Autodesk Fusion 360 part; units mm, degrees
(part 7 of 9)
sketch "草图25" plane through (0, -82, 0) normal (0, 1, 0) x (-1, 0, 0)
  line L0 (41, 0) -> (116, 0)
  line L1 (116, 0) -> (116, 140)
  line L2 (116, 140) -> (41, 140)
  line L3 (41, 140) -> (41, 0)
  line L4 (53.0801, 20.799) -> (48.75, 18.299)
  line L5 (48.75, 18.299) -> (48.75, 13.299)
  line L6 (48.75, 13.299) -> (53.0801, 10.799)
  line L7 (53.0801, 10.799) -> (57.4103, 13.299)
  line L8 (57.4103, 13.299) -> (57.4103, 18.299)
  line L9 (57.4103, 18.299) -> (53.0801, 20.799)
  line L10 (63.2404, 20.799) -> (58.9103, 18.299)
  line L11 (58.9103, 18.299) -> (58.9103, 13.299)
  line L12 (58.9103, 13.299) -> (63.2404, 10.799)
  line L13 (63.2404, 10.799) -> (67.5705, 13.299)
  line L14 (67.5705, 13.299) -> (67.5705, 18.299)
  line L15 (67.5705, 18.299) -> (63.2404, 20.799)
  line L16 (73.4006, 20.799) -> (69.0705, 18.299)
  line L17 (69.0705, 18.299) -> (69.0705, 13.299)
  line L18 (69.0705, 13.299) -> (73.4006, 10.799)
  line L19 (73.4006, 10.799) -> (77.7308, 13.299)
  line L20 (77.7308, 13.299) -> (77.7308, 18.299)
  line L21 (77.7308, 18.299) -> (73.4006, 20.799)
  line L22 (83.5609, 20.799) -> (79.2308, 18.299)
  line L23 (79.2308, 18.299) -> (79.2308, 13.299)
  line L24 (79.2308, 13.299) -> (83.5609, 10.799)
  line L25 (83.5609, 10.799) -> (87.891, 13.299)
  line L26 (87.891, 13.299) -> (87.891, 18.299)
  line L27 (87.891, 18.299) -> (83.5609, 20.799)
  line L28 (93.7211, 20.799) -> (89.391, 18.299)
  line L29 (89.391, 18.299) -> (89.391, 13.299)
  line L30 (89.391, 13.299) -> (93.7211, 10.799)
  line L31 (93.7211, 10.799) -> (98.0513, 13.299)
  line L32 (98.0513, 13.299) -> (98.0513, 18.299)
  line L33 (98.0513, 18.299) -> (93.7211, 20.799)
  line L34 (103.8814, 20.799) -> (99.5513, 18.299)
  line L35 (99.5513, 18.299) -> (99.5513, 13.299)
  line L36 (99.5513, 13.299) -> (103.8814, 10.799)
  line L37 (103.8814, 10.799) -> (108.2115, 13.299)
  line L38 (108.2115, 13.299) -> (108.2115, 18.299)
  line L39 (108.2115, 18.299) -> (103.8814, 20.799)
  line L40 (48, 29.5981) -> (43.6699, 27.0981)
  line L41 (43.6699, 27.0981) -> (43.6699, 22.0981)
  line L42 (43.6699, 22.0981) -> (48, 19.5981)
  line L43 (48, 19.5981) -> (52.3301, 22.0981)
  line L44 (52.3301, 22.0981) -> (52.3301, 27.0981)
  line L45 (52.3301, 27.0981) -> (48, 29.5981)
  line L46 (58.1603, 29.5981) -> (53.8301, 27.0981)
  line L47 (53.8301, 27.0981) -> (53.8301, 22.0981)
  line L48 (53.8301, 22.0981) -> (58.1603, 19.5981)
  line L49 (58.1603, 19.5981) -> (62.4904, 22.0981)
  line L50 (62.4904, 22.0981) -> (62.4904, 27.0981)
  line L51 (62.4904, 27.0981) -> (58.1603, 29.5981)
  line L52 (68.3205, 29.5981) -> (63.9904, 27.0981)
  line L53 (63.9904, 27.0981) -> (63.9904, 22.0981)
  line L54 (63.9904, 22.0981) -> (68.3205, 19.5981)
  line L55 (68.3205, 19.5981) -> (72.6506, 22.0981)
  line L56 (72.6506, 22.0981) -> (72.6506, 27.0981)
  line L57 (72.6506, 27.0981) -> (68.3205, 29.5981)
  line L58 (78.4808, 29.5981) -> (74.1506, 27.0981)
  line L59 (74.1506, 27.0981) -> (74.1506, 22.0981)
  line L60 (74.1506, 22.0981) -> (78.4808, 19.5981)
  line L61 (78.4808, 19.5981) -> (82.8109, 22.0981)
  line L62 (82.8109, 22.0981) -> (82.8109, 27.0981)
  line L63 (82.8109, 27.0981) -> (78.4808, 29.5981)
  line L64 (88.641, 29.5981) -> (84.3109, 27.0981)
  line L65 (84.3109, 27.0981) -> (84.3109, 22.0981)
  line L66 (84.3109, 22.0981) -> (88.641, 19.5981)
  line L67 (88.641, 19.5981) -> (92.9711, 22.0981)
  line L68 (92.9711, 22.0981) -> (92.9711, 27.0981)
  line L69 (92.9711, 27.0981) -> (88.641, 29.5981)
  line L70 (98.8013, 29.5981) -> (94.4711, 27.0981)
  line L71 (94.4711, 27.0981) -> (94.4711, 22.0981)
  line L72 (94.4711, 22.0981) -> (98.8013, 19.5981)
  line L73 (98.8013, 19.5981) -> (103.1314, 22.0981)
  line L74 (103.1314, 22.0981) -> (103.1314, 27.0981)
  line L75 (103.1314, 27.0981) -> (98.8013, 29.5981)
  line L76 (108.9615, 29.5981) -> (104.6314, 27.0981)
  line L77 (104.6314, 27.0981) -> (104.6314, 22.0981)
  line L78 (104.6314, 22.0981) -> (108.9615, 19.5981)
  line L79 (108.9615, 19.5981) -> (113.2917, 22.0981)
  line L80 (113.2917, 22.0981) -> (113.2917, 27.0981)
  line L81 (113.2917, 27.0981) -> (108.9615, 29.5981)
  line L82 (53.0801, 38.3971) -> (48.75, 35.8971)
  line L83 (48.75, 35.8971) -> (48.75, 30.8971)
  line L84 (48.75, 30.8971) -> (53.0801, 28.3971)
  line L85 (53.0801, 28.3971) -> (57.4103, 30.8971)
  line L86 (57.4103, 30.8971) -> (57.4103, 35.8971)
  line L87 (57.4103, 35.8971) -> (53.0801, 38.3971)
  line L88 (63.2404, 38.3971) -> (58.9103, 35.8971)
  line L89 (58.9103, 35.8971) -> (58.9103, 30.8971)
  line L90 (58.9103, 30.8971) -> (63.2404, 28.3971)
  line L91 (63.2404, 28.3971) -> (67.5705, 30.8971)
  line L92 (67.5705, 30.8971) -> (67.5705, 35.8971)
  line L93 (67.5705, 35.8971) -> (63.2404, 38.3971)
  line L94 (73.4006, 38.3971) -> (69.0705, 35.8971)
  line L95 (69.0705, 35.8971) -> (69.0705, 30.8971)
  line L96 (69.0705, 30.8971) -> (73.4006, 28.3971)
  line L97 (73.4006, 28.3971) -> (77.7308, 30.8971)
  line L98 (77.7308, 30.8971) -> (77.7308, 35.8971)
  line L99 (77.7308, 35.8971) -> (73.4006, 38.3971)
  line L100 (83.5609, 38.3971) -> (79.2308, 35.8971)
  line L101 (79.2308, 35.8971) -> (79.2308, 30.8971)
  line L102 (79.2308, 30.8971) -> (83.5609, 28.3971)
  line L103 (83.5609, 28.3971) -> (87.891, 30.8971)
  line L104 (87.891, 30.8971) -> (87.891, 35.8971)
  line L105 (87.891, 35.8971) -> (83.5609, 38.3971)
  line L106 (93.7211, 38.3971) -> (89.391, 35.8971)
  line L107 (89.391, 35.8971) -> (89.391, 30.8971)
  line L108 (89.391, 30.8971) -> (93.7211, 28.3971)
  line L109 (93.7211, 28.3971) -> (98.0513, 30.8971)
  line L110 (98.0513, 30.8971) -> (98.0513, 35.8971)
  line L111 (98.0513, 35.8971) -> (93.7211, 38.3971)
  line L112 (103.8814, 38.3971) -> (99.5513, 35.8971)
  line L113 (99.5513, 35.8971) -> (99.5513, 30.8971)
  line L114 (99.5513, 30.8971) -> (103.8814, 28.3971)
  line L115 (103.8814, 28.3971) -> (108.2115, 30.8971)
  line L116 (108.2115, 30.8971) -> (108.2115, 35.8971)
  line L117 (108.2115, 35.8971) -> (103.8814, 38.3971)
  line L118 (48, 47.1962) -> (43.6699, 44.6962)
  line L119 (43.6699, 44.6962) -> (43.6699, 39.6962)
  line L120 (43.6699, 39.6962) -> (48, 37.1962)
  line L121 (48, 37.1962) -> (52.3301, 39.6962)
  line L122 (52.3301, 39.6962) -> (52.3301, 44.6962)
  line L123 (52.3301, 44.6962) -> (48, 47.1962)
  line L124 (58.1603, 47.1962) -> (53.8301, 44.6962)
  line L125 (53.8301, 44.6962) -> (53.8301, 39.6962)
  line L126 (53.8301, 39.6962) -> (58.1603, 37.1962)
  line L127 (58.1603, 37.1962) -> (62.4904, 39.6962)
  line L128 (62.4904, 39.6962) -> (62.4904, 44.6962)
  line L129 (62.4904, 44.6962) -> (58.1603, 47.1962)
  line L130 (68.3205, 47.1962) -> (63.9904, 44.6962)
  line L131 (63.9904, 44.6962) -> (63.9904, 39.6962)
  line L132 (63.9904, 39.6962) -> (68.3205, 37.1962)
  line L133 (68.3205, 37.1962) -> (72.6506, 39.6962)
  line L134 (72.6506, 39.6962) -> (72.6506, 44.6962)
  line L135 (72.6506, 44.6962) -> (68.3205, 47.1962)
  line L136 (78.4808, 47.1962) -> (74.1506, 44.6962)
  line L137 (74.1506, 44.6962) -> (74.1506, 39.6962)
  line L138 (74.1506, 39.6962) -> (78.4808, 37.1962)
  line L139 (78.4808, 37.1962) -> (82.8109, 39.6962)
  line L140 (82.8109, 39.6962) -> (82.8109, 44.6962)
  line L141 (82.8109, 44.6962) -> (78.4808, 47.1962)
  line L142 (88.641, 47.1962) -> (84.3109, 44.6962)
  line L143 (84.3109, 44.6962) -> (84.3109, 39.6962)
  line L144 (84.3109, 39.6962) -> (88.641, 37.1962)
  line L145 (88.641, 37.1962) -> (92.9711, 39.6962)
  line L146 (92.9711, 39.6962) -> (92.9711, 44.6962)
  line L147 (92.9711, 44.6962) -> (88.641, 47.1962)
  line L148 (98.8013, 47.1962) -> (94.4711, 44.6962)
  line L149 (94.4711, 44.6962) -> (94.4711, 39.6962)
  line L150 (94.4711, 39.6962) -> (98.8013, 37.1962)
  line L151 (98.8013, 37.1962) -> (103.1314, 39.6962)
  line L152 (103.1314, 39.6962) -> (103.1314, 44.6962)
  line L153 (103.1314, 44.6962) -> (98.8013, 47.1962)
  line L154 (108.9615, 47.1962) -> (104.6314, 44.6962)
  line L155 (104.6314, 44.6962) -> (104.6314, 39.6962)
  line L156 (104.6314, 39.6962) -> (108.9615, 37.1962)
  line L157 (108.9615, 37.1962) -> (113.2917, 39.6962)
  line L158 (113.2917, 39.6962) -> (113.2917, 44.6962)
  line L159 (113.2917, 44.6962) -> (108.9615, 47.1962)
  line L160 (53.0801, 55.9952) -> (48.75, 53.4952)
  line L161 (48.75, 53.4952) -> (48.75, 48.4952)
  line L162 (48.75, 48.4952) -> (53.0801, 45.9952)
  line L163 (53.0801, 45.9952) -> (57.4103, 48.4952)
  line L164 (57.4103, 48.4952) -> (57.4103, 53.4952)
  line L165 (57.4103, 53.4952) -> (53.0801, 55.9952)
  line L166 (63.2404, 55.9952) -> (58.9103, 53.4952)
  line L167 (58.9103, 53.4952) -> (58.9103, 48.4952)
  line L168 (58.9103, 48.4952) -> (63.2404, 45.9952)
  line L169 (63.2404, 45.9952) -> (67.5705, 48.4952)
  line L170 (67.5705, 48.4952) -> (67.5705, 53.4952)
  line L171 (67.5705, 53.4952) -> (63.2404, 55.9952)
  line L172 (73.4006, 55.9952) -> (69.0705, 53.4952)
  line L173 (69.0705, 53.4952) -> (69.0705, 48.4952)
  line L174 (69.0705, 48.4952) -> (73.4006, 45.9952)
  line L175 (73.4006, 45.9952) -> (77.7308, 48.4952)
  line L176 (77.7308, 48.4952) -> (77.7308, 53.4952)
  line L177 (77.7308, 53.4952) -> (73.4006, 55.9952)
  line L178 (83.5609, 55.9952) -> (79.2308, 53.4952)
  line L179 (79.2308, 53.4952) -> (79.2308, 48.4952)
  line L180 (79.2308, 48.4952) -> (83.5609, 45.9952)
  line L181 (83.5609, 45.9952) -> (87.891, 48.4952)
  line L182 (87.891, 48.4952) -> (87.891, 53.4952)
  line L183 (87.891, 53.4952) -> (83.5609, 55.9952)
  line L184 (93.7211, 55.9952) -> (89.391, 53.4952)
  line L185 (89.391, 53.4952) -> (89.391, 48.4952)
  line L186 (89.391, 48.4952) -> (93.7211, 45.9952)
  line L187 (93.7211, 45.9952) -> (98.0513, 48.4952)
  line L188 (98.0513, 48.4952) -> (98.0513, 53.4952)
  line L189 (98.0513, 53.4952) -> (93.7211, 55.9952)
  line L190 (103.8814, 55.9952) -> (99.5513, 53.4952)
  line L191 (99.5513, 53.4952) -> (99.5513, 48.4952)
  line L192 (99.5513, 48.4952) -> (103.8814, 45.9952)
  line L193 (103.8814, 45.9952) -> (108.2115, 48.4952)
  line L194 (108.2115, 48.4952) -> (108.2115, 53.4952)
  line L195 (108.2115, 53.4952) -> (103.8814, 55.9952)
  line L196 (48, 64.7942) -> (43.6699, 62.2942)
  line L197 (43.6699, 62.2942) -> (43.6699, 57.2942)
  line L198 (43.6699, 57.2942) -> (48, 54.7942)
  line L199 (48, 54.7942) -> (52.3301, 57.2942)
  line L200 (52.3301, 57.2942) -> (52.3301, 62.2942)
  line L201 (52.3301, 62.2942) -> (48, 64.7942)
  line L202 (58.1603, 64.7942) -> (53.8301, 62.2942)
  line L203 (53.8301, 62.2942) -> (53.8301, 57.2942)
  line L204 (53.8301, 57.2942) -> (58.1603, 54.7942)
  line L205 (58.1603, 54.7942) -> (62.4904, 57.2942)
  line L206 (62.4904, 57.2942) -> (62.4904, 62.2942)
  line L207 (62.4904, 62.2942) -> (58.1603, 64.7942)
  line L208 (68.3205, 64.7942) -> (63.9904, 62.2942)
  line L209 (63.9904, 62.2942) -> (63.9904, 57.2942)
  line L210 (63.9904, 57.2942) -> (68.3205, 54.7942)
  line L211 (68.3205, 54.7942) -> (72.6506, 57.2942)
  line L212 (72.6506, 57.2942) -> (72.6506, 62.2942)
  line L213 (72.6506, 62.2942) -> (68.3205, 64.7942)
  line L214 (78.4808, 64.7942) -> (74.1506, 62.2942)
  line L215 (74.1506, 62.2942) -> (74.1506, 57.2942)
  line L216 (74.1506, 57.2942) -> (78.4808, 54.7942)
  line L217 (78.4808, 54.7942) -> (82.8109, 57.2942)
  line L218 (82.8109, 57.2942) -> (82.8109, 62.2942)
  line L219 (82.8109, 62.2942) -> (78.4808, 64.7942)
  line L220 (88.641, 64.7942) -> (84.3109, 62.2942)
  line L221 (84.3109, 62.2942) -> (84.3109, 57.2942)
  line L222 (84.3109, 57.2942) -> (88.641, 54.7942)
  line L223 (88.641, 54.7942) -> (92.9711, 57.2942)
  line L224 (92.9711, 57.2942) -> (92.9711, 62.2942)
  line L225 (92.9711, 62.2942) -> (88.641, 64.7942)
  line L226 (98.8013, 64.7942) -> (94.4711, 62.2942)
  line L227 (94.4711, 62.2942) -> (94.4711, 57.2942)
  line L228 (94.4711, 57.2942) -> (98.8013, 54.7942)
  line L229 (98.8013, 54.7942) -> (103.1314, 57.2942)
  line L230 (103.1314, 57.2942) -> (103.1314, 62.2942)
  line L231 (103.1314, 62.2942) -> (98.8013, 64.7942)
  line L232 (108.9615, 64.7942) -> (104.6314, 62.2942)
  line L233 (104.6314, 62.2942) -> (104.6314, 57.2942)
  line L234 (104.6314, 57.2942) -> (108.9615, 54.7942)
  line L235 (108.9615, 54.7942) -> (113.2917, 57.2942)
  line L236 (113.2917, 57.2942) -> (113.2917, 62.2942)
  line L237 (113.2917, 62.2942) -> (108.9615, 64.7942)
  line L238 (53.0801, 73.5933) -> (48.75, 71.0933)
  line L239 (48.75, 71.0933) -> (48.75, 66.0933)
  line L240 (48.75, 66.0933) -> (53.0801, 63.5933)
  line L241 (53.0801, 63.5933) -> (57.4103, 66.0933)
  line L242 (57.4103, 66.0933) -> (57.4103, 71.0933)
  line L243 (57.4103, 71.0933) -> (53.0801, 73.5933)
  line L244 (63.2404, 73.5933) -> (58.9103, 71.0933)
  line L245 (58.9103, 71.0933) -> (58.9103, 66.0933)
  line L246 (58.9103, 66.0933) -> (63.2404, 63.5933)
  line L247 (63.2404, 63.5933) -> (67.5705, 66.0933)
  line L248 (67.5705, 66.0933) -> (67.5705, 71.0933)
  line L249 (67.5705, 71.0933) -> (63.2404, 73.5933)
  line L250 (73.4006, 73.5933) -> (69.0705, 71.0933)
  line L251 (69.0705, 71.0933) -> (69.0705, 66.0933)
  line L252 (69.0705, 66.0933) -> (73.4006, 63.5933)
  line L253 (73.4006, 63.5933) -> (77.7308, 66.0933)
  line L254 (77.7308, 66.0933) -> (77.7308, 71.0933)
  line L255 (77.7308, 71.0933) -> (73.4006, 73.5933)
  line L256 (83.5609, 73.5933) -> (79.2308, 71.0933)
  line L257 (79.2308, 71.0933) -> (79.2308, 66.0933)
  line L258 (79.2308, 66.0933) -> (83.5609, 63.5933)
  line L259 (83.5609, 63.5933) -> (87.891, 66.0933)
  line L260 (87.891, 66.0933) -> (87.891, 71.0933)
  line L261 (87.891, 71.0933) -> (83.5609, 73.5933)
  line L262 (93.7211, 73.5933) -> (89.391, 71.0933)
  line L263 (89.391, 71.0933) -> (89.391, 66.0933)
  line L264 (89.391, 66.0933) -> (93.7211, 63.5933)
  line L265 (93.7211, 63.5933) -> (98.0513, 66.0933)
  line L266 (98.0513, 66.0933) -> (98.0513, 71.0933)
  line L267 (98.0513, 71.0933) -> (93.7211, 73.5933)
  line L268 (103.8814, 73.5933) -> (99.5513, 71.0933)
  line L269 (99.5513, 71.0933) -> (99.5513, 66.0933)
  line L270 (99.5513, 66.0933) -> (103.8814, 63.5933)
  line L271 (103.8814, 63.5933) -> (108.2115, 66.0933)
  line L272 (108.2115, 66.0933) -> (108.2115, 71.0933)
  line L273 (108.2115, 71.0933) -> (103.8814, 73.5933)
  line L274 (48, 82.3923) -> (43.6699, 79.8923)
  line L275 (43.6699, 79.8923) -> (43.6699, 74.8923)
  line L276 (43.6699, 74.8923) -> (48, 72.3923)
  line L277 (48, 72.3923) -> (52.3301, 74.8923)
  line L278 (52.3301, 74.8923) -> (52.3301, 79.8923)
  line L279 (52.3301, 79.8923) -> (48, 82.3923)
  line L280 (58.1603, 82.3923) -> (53.8301, 79.8923)
  line L281 (53.8301, 79.8923) -> (53.8301, 74.8923)
  line L282 (53.8301, 74.8923) -> (58.1603, 72.3923)
  line L283 (58.1603, 72.3923) -> (62.4904, 74.8923)
  line L284 (62.4904, 74.8923) -> (62.4904, 79.8923)
  line L285 (62.4904, 79.8923) -> (58.1603, 82.3923)
  line L286 (68.3205, 82.3923) -> (63.9904, 79.8923)
  line L287 (63.9904, 79.8923) -> (63.9904, 74.8923)
  line L288 (63.9904, 74.8923) -> (68.3205, 72.3923)
  line L289 (68.3205, 72.3923) -> (72.6506, 74.8923)
  line L290 (72.6506, 74.8923) -> (72.6506, 79.8923)
  line L291 (72.6506, 79.8923) -> (68.3205, 82.3923)
  line L292 (78.4808, 82.3923) -> (74.1506, 79.8923)
  line L293 (74.1506, 79.8923) -> (74.1506, 74.8923)
  line L294 (74.1506, 74.8923) -> (78.4808, 72.3923)
  line L295 (78.4808, 72.3923) -> (82.8109, 74.8923)
  line L296 (82.8109, 74.8923) -> (82.8109, 79.8923)
  line L297 (82.8109, 79.8923) -> (78.4808, 82.3923)
  line L298 (88.641, 82.3923) -> (84.3109, 79.8923)
  line L299 (84.3109, 79.8923) -> (84.3109, 74.8923)
  line L300 (84.3109, 74.8923) -> (88.641, 72.3923)
  line L301 (88.641, 72.3923) -> (92.9711, 74.8923)
  line L302 (92.9711, 74.8923) -> (92.9711, 79.8923)
  line L303 (92.9711, 79.8923) -> (88.641, 82.3923)
  line L304 (98.8013, 82.3923) -> (94.4711, 79.8923)
  line L305 (94.4711, 79.8923) -> (94.4711, 74.8923)
  line L306 (94.4711, 74.8923) -> (98.8013, 72.3923)
  line L307 (98.8013, 72.3923) -> (103.1314, 74.8923)
  line L308 (103.1314, 74.8923) -> (103.1314, 79.8923)
  line L309 (103.1314, 79.8923) -> (98.8013, 82.3923)
  line L310 (108.9615, 82.3923) -> (104.6314, 79.8923)
  line L311 (104.6314, 79.8923) -> (104.6314, 74.8923)
  line L312 (104.6314, 74.8923) -> (108.9615, 72.3923)
  line L313 (108.9615, 72.3923) -> (113.2917, 74.8923)
  line L314 (113.2917, 74.8923) -> (113.2917, 79.8923)
  line L315 (113.2917, 79.8923) -> (108.9615, 82.3923)
  line L316 (53.0801, 91.1913) -> (48.75, 88.6913)
  line L317 (48.75, 88.6913) -> (48.75, 83.6913)
  line L318 (48.75, 83.6913) -> (53.0801, 81.1913)
  line L319 (53.0801, 81.1913) -> (57.4103, 83.6913)
  line L320 (57.4103, 83.6913) -> (57.4103, 88.6913)
  line L321 (57.4103, 88.6913) -> (53.0801, 91.1913)
  line L322 (63.2404, 91.1913) -> (58.9103, 88.6913)
  line L323 (58.9103, 88.6913) -> (58.9103, 83.6913)
  line L324 (58.9103, 83.6913) -> (63.2404, 81.1913)
  line L325 (63.2404, 81.1913) -> (67.5705, 83.6913)
  line L326 (67.5705, 83.6913) -> (67.5705, 88.6913)
  line L327 (67.5705, 88.6913) -> (63.2404, 91.1913)
  line L328 (73.4006, 91.1913) -> (69.0705, 88.6913)
  line L329 (69.0705, 88.6913) -> (69.0705, 83.6913)
  line L330 (69.0705, 83.6913) -> (73.4006, 81.1913)
  line L331 (73.4006, 81.1913) -> (77.7308, 83.6913)
  line L332 (77.7308, 83.6913) -> (77.7308, 88.6913)
  line L333 (77.7308, 88.6913) -> (73.4006, 91.1913)
  line L334 (83.5609, 91.1913) -> (79.2308, 88.6913)
  line L335 (79.2308, 88.6913) -> (79.2308, 83.6913)
  line L336 (79.2308, 83.6913) -> (83.5609, 81.1913)
  line L337 (83.5609, 81.1913) -> (87.891, 83.6913)
  line L338 (87.891, 83.6913) -> (87.891, 88.6913)
  line L339 (87.891, 88.6913) -> (83.5609, 91.1913)
  line L340 (93.7211, 91.1913) -> (89.391, 88.6913)
  line L341 (89.391, 88.6913) -> (89.391, 83.6913)
  line L342 (89.391, 83.6913) -> (93.7211, 81.1913)
  line L343 (93.7211, 81.1913) -> (98.0513, 83.6913)
  line L344 (98.0513, 83.6913) -> (98.0513, 88.6913)
  line L345 (98.0513, 88.6913) -> (93.7211, 91.1913)
  line L346 (103.8814, 91.1913) -> (99.5513, 88.6913)
  line L347 (99.5513, 88.6913) -> (99.5513, 83.6913)
  line L348 (99.5513, 83.6913) -> (103.8814, 81.1913)
  line L349 (103.8814, 81.1913) -> (108.2115, 83.6913)
  line L350 (108.2115, 83.6913) -> (108.2115, 88.6913)
  line L351 (108.2115, 88.6913) -> (103.8814, 91.1913)
  line L352 (48, 99.9904) -> (43.6699, 97.4904)
  line L353 (43.6699, 97.4904) -> (43.6699, 92.4904)
  line L354 (43.6699, 92.4904) -> (48, 89.9904)
  line L355 (48, 89.9904) -> (52.3301, 92.4904)
  line L356 (52.3301, 92.4904) -> (52.3301, 97.4904)
  line L357 (52.3301, 97.4904) -> (48, 99.9904)
  line L358 (58.1603, 99.9904) -> (53.8301, 97.4904)
  line L359 (53.8301, 97.4904) -> (53.8301, 92.4904)
  line L360 (53.8301, 92.4904) -> (58.1603, 89.9904)
  line L361 (58.1603, 89.9904) -> (62.4904, 92.4904)
  line L362 (62.4904, 92.4904) -> (62.4904, 97.4904)
  line L363 (62.4904, 97.4904) -> (58.1603, 99.9904)
  line L364 (68.3205, 99.9904) -> (63.9904, 97.4904)
  line L365 (63.9904, 97.4904) -> (63.9904, 92.4904)
  line L366 (63.9904, 92.4904) -> (68.3205, 89.9904)
  line L367 (68.3205, 89.9904) -> (72.6506, 92.4904)
  line L368 (72.6506, 92.4904) -> (72.6506, 97.4904)
  line L369 (72.6506, 97.4904) -> (68.3205, 99.9904)
  line L370 (78.4808, 99.9904) -> (74.1506, 97.4904)
  line L371 (74.1506, 97.4904) -> (74.1506, 92.4904)
  line L372 (74.1506, 92.4904) -> (78.4808, 89.9904)
  line L373 (78.4808, 89.9904) -> (82.8109, 92.4904)
  line L374 (82.8109, 92.4904) -> (82.8109, 97.4904)
  line L375 (82.8109, 97.4904) -> (78.4808, 99.9904)
  line L376 (88.641, 99.9904) -> (84.3109, 97.4904)
  line L377 (84.3109, 97.4904) -> (84.3109, 92.4904)
  line L378 (84.3109, 92.4904) -> (88.641, 89.9904)
  line L379 (88.641, 89.9904) -> (92.9711, 92.4904)
  line L380 (92.9711, 92.4904) -> (92.9711, 97.4904)
  line L381 (92.9711, 97.4904) -> (88.641, 99.9904)
  line L382 (98.8013, 99.9904) -> (94.4711, 97.4904)
  line L383 (94.4711, 97.4904) -> (94.4711, 92.4904)
  line L384 (94.4711, 92.4904) -> (98.8013, 89.9904)
  line L385 (98.8013, 89.9904) -> (103.1314, 92.4904)
  line L386 (103.1314, 92.4904) -> (103.1314, 97.4904)
  line L387 (103.1314, 97.4904) -> (98.8013, 99.9904)
  line L388 (108.9615, 99.9904) -> (104.6314, 97.4904)
  line L389 (104.6314, 97.4904) -> (104.6314, 92.4904)
  line L390 (104.6314, 92.4904) -> (108.9615, 89.9904)
  line L391 (108.9615, 89.9904) -> (113.2917, 92.4904)
  line L392 (113.2917, 92.4904) -> (113.2917, 97.4904)
  line L393 (113.2917, 97.4904) -> (108.9615, 99.9904)
  line L394 (53.0801, 108.7894) -> (48.75, 106.2894)
  line L395 (48.75, 106.2894) -> (48.75, 101.2894)
  line L396 (48.75, 101.2894) -> (53.0801, 98.7894)
  line L397 (53.0801, 98.7894) -> (57.4103, 101.2894)
  line L398 (57.4103, 101.2894) -> (57.4103, 106.2894)
  line L399 (57.4103, 106.2894) -> (53.0801, 108.7894)
  line L400 (63.2404, 108.7894) -> (58.9103, 106.2894)
  line L401 (58.9103, 106.2894) -> (58.9103, 101.2894)
  line L402 (58.9103, 101.2894) -> (63.2404, 98.7894)
  line L403 (63.2404, 98.7894) -> (67.5705, 101.2894)
  line L404 (67.5705, 101.2894) -> (67.5705, 106.2894)
  line L405 (67.5705, 106.2894) -> (63.2404, 108.7894)
  line L406 (73.4006, 108.7894) -> (69.0705, 106.2894)
  line L407 (69.0705, 106.2894) -> (69.0705, 101.2894)
  line L408 (69.0705, 101.2894) -> (73.4006, 98.7894)
  line L409 (73.4006, 98.7894) -> (77.7308, 101.2894)
  line L410 (77.7308, 101.2894) -> (77.7308, 106.2894)
  line L411 (77.7308, 106.2894) -> (73.4006, 108.7894)
  line L412 (83.5609, 108.7894) -> (79.2308, 106.2894)
  line L413 (79.2308, 106.2894) -> (79.2308, 101.2894)
  line L414 (79.2308, 101.2894) -> (83.5609, 98.7894)
  line L415 (83.5609, 98.7894) -> (87.891, 101.2894)
  line L416 (87.891, 101.2894) -> (87.891, 106.2894)
  line L417 (87.891, 106.2894) -> (83.5609, 108.7894)
  line L418 (93.7211, 108.7894) -> (89.391, 106.2894)
  line L419 (89.391, 106.2894) -> (89.391, 101.2894)
  line L420 (89.391, 101.2894) -> (93.7211, 98.7894)
  line L421 (93.7211, 98.7894) -> (98.0513, 101.2894)
  line L422 (98.0513, 101.2894) -> (98.0513, 106.2894)
  line L423 (98.0513, 106.2894) -> (93.7211, 108.7894)
  line L424 (103.8814, 108.7894) -> (99.5513, 106.2894)
  line L425 (99.5513, 106.2894) -> (99.5513, 101.2894)
  line L426 (99.5513, 101.2894) -> (103.8814, 98.7894)
  line L427 (103.8814, 98.7894) -> (108.2115, 101.2894)
  line L428 (108.2115, 101.2894) -> (108.2115, 106.2894)
  line L429 (108.2115, 106.2894) -> (103.8814, 108.7894)
  line L430 (48, 117.5885) -> (43.6699, 115.0885)
  line L431 (43.6699, 115.0885) -> (43.6699, 110.0885)
  line L432 (43.6699, 110.0885) -> (48, 107.5885)
  line L433 (48, 107.5885) -> (52.3301, 110.0885)
  line L434 (52.3301, 110.0885) -> (52.3301, 115.0885)
  line L435 (52.3301, 115.0885) -> (48, 117.5885)
  line L436 (58.1603, 117.5885) -> (53.8301, 115.0885)
  line L437 (53.8301, 115.0885) -> (53.8301, 110.0885)
  line L438 (53.8301, 110.0885) -> (58.1603, 107.5885)
  line L439 (58.1603, 107.5885) -> (62.4904, 110.0885)
  line L440 (62.4904, 110.0885) -> (62.4904, 115.0885)
  line L441 (62.4904, 115.0885) -> (58.1603, 117.5885)
  line L442 (68.3205, 117.5885) -> (63.9904, 115.0885)
  line L443 (63.9904, 115.0885) -> (63.9904, 110.0885)
  line L444 (63.9904, 110.0885) -> (68.3205, 107.5885)
  line L445 (68.3205, 107.5885) -> (72.6506, 110.0885)
  line L446 (72.6506, 110.0885) -> (72.6506, 115.0885)
  line L447 (72.6506, 115.0885) -> (68.3205, 117.5885)
  line L448 (78.4808, 117.5885) -> (74.1506, 115.0885)
  line L449 (74.1506, 115.0885) -> (74.1506, 110.0885)
  line L450 (74.1506, 110.0885) -> (78.4808, 107.5885)
  line L451 (78.4808, 107.5885) -> (82.8109, 110.0885)
  line L452 (82.8109, 110.0885) -> (82.8109, 115.0885)
  line L453 (82.8109, 115.0885) -> (78.4808, 117.5885)
  line L454 (88.641, 117.5885) -> (84.3109, 115.0885)
  line L455 (84.3109, 115.0885) -> (84.3109, 110.0885)
  line L456 (84.3109, 110.0885) -> (88.641, 107.5885)
  line L457 (88.641, 107.5885) -> (92.9711, 110.0885)
  line L458 (92.9711, 110.0885) -> (92.9711, 115.0885)
  line L459 (92.9711, 115.0885) -> (88.641, 117.5885)
  line L460 (98.8013, 117.5885) -> (94.4711, 115.0885)
  line L461 (94.4711, 115.0885) -> (94.4711, 110.0885)
  line L462 (94.4711, 110.0885) -> (98.8013, 107.5885)
  line L463 (98.8013, 107.5885) -> (103.1314, 110.0885)
  line L464 (103.1314, 110.0885) -> (103.1314, 115.0885)
  line L465 (103.1314, 115.0885) -> (98.8013, 117.5885)
  line L466 (108.9615, 117.5885) -> (104.6314, 115.0885)
  line L467 (104.6314, 115.0885) -> (104.6314, 110.0885)
  line L468 (104.6314, 110.0885) -> (108.9615, 107.5885)
  line L469 (108.9615, 107.5885) -> (113.2917, 110.0885)
  line L470 (113.2917, 110.0885) -> (113.2917, 115.0885)
  line L471 (113.2917, 115.0885) -> (108.9615, 117.5885)
  line L472 (53.0801, 126.3875) -> (48.75, 123.8875)
  line L473 (48.75, 123.8875) -> (48.75, 118.8875)
  line L474 (48.75, 118.8875) -> (53.0801, 116.3875)
  line L475 (53.0801, 116.3875) -> (57.4103, 118.8875)
  line L476 (57.4103, 118.8875) -> (57.4103, 123.8875)
  line L477 (57.4103, 123.8875) -> (53.0801, 126.3875)
  line L478 (63.2404, 126.3875) -> (58.9103, 123.8875)
  line L479 (58.9103, 123.8875) -> (58.9103, 118.8875)
  line L480 (58.9103, 118.8875) -> (63.2404, 116.3875)
  line L481 (63.2404, 116.3875) -> (67.5705, 118.8875)
  line L482 (67.5705, 118.8875) -> (67.5705, 123.8875)
  line L483 (67.5705, 123.8875) -> (63.2404, 126.3875)
  line L484 (73.4006, 126.3875) -> (69.0705, 123.8875)
  line L485 (69.0705, 123.8875) -> (69.0705, 118.8875)
  line L486 (69.0705, 118.8875) -> (73.4006, 116.3875)
  line L487 (73.4006, 116.3875) -> (77.7308, 118.8875)
  line L488 (77.7308, 118.8875) -> (77.7308, 123.8875)
  line L489 (77.7308, 123.8875) -> (73.4006, 126.3875)
  line L490 (83.5609, 126.3875) -> (79.2308, 123.8875)
  line L491 (79.2308, 123.8875) -> (79.2308, 118.8875)
  line L492 (79.2308, 118.8875) -> (83.5609, 116.3875)
  line L493 (83.5609, 116.3875) -> (87.891, 118.8875)
  line L494 (87.891, 118.8875) -> (87.891, 123.8875)
  line L495 (87.891, 123.8875) -> (83.5609, 126.3875)
  line L496 (93.7211, 126.3875) -> (89.391, 123.8875)
  line L497 (89.391, 123.8875) -> (89.391, 118.8875)
  line L498 (89.391, 118.8875) -> (93.7211, 116.3875)
  line L499 (93.7211, 116.3875) -> (98.0513, 118.8875)
  line L500 (98.0513, 118.8875) -> (98.0513, 123.8875)
  line L501 (98.0513, 123.8875) -> (93.7211, 126.3875)
  line L502 (103.8814, 126.3875) -> (99.5513, 123.8875)
  line L503 (99.5513, 123.8875) -> (99.5513, 118.8875)
  line L504 (99.5513, 118.8875) -> (103.8814, 116.3875)
  line L505 (103.8814, 116.3875) -> (108.2115, 118.8875)
  line L506 (108.2115, 118.8875) -> (108.2115, 123.8875)
  line L507 (108.2115, 123.8875) -> (103.8814, 126.3875)
  line L508 (48, 135.1865) -> (43.6699, 132.6865)
  line L509 (43.6699, 132.6865) -> (43.6699, 127.6865)
  line L510 (43.6699, 127.6865) -> (48, 125.1865)
  line L511 (48, 125.1865) -> (52.3301, 127.6865)
  line L512 (52.3301, 127.6865) -> (52.3301, 132.6865)
  line L513 (52.3301, 132.6865) -> (48, 135.1865)
  line L514 (58.1603, 135.1865) -> (53.8301, 132.6865)
  line L515 (53.8301, 132.6865) -> (53.8301, 127.6865)
  line L516 (53.8301, 127.6865) -> (58.1603, 125.1865)
  line L517 (58.1603, 125.1865) -> (62.4904, 127.6865)
  line L518 (62.4904, 127.6865) -> (62.4904, 132.6865)
  line L519 (62.4904, 132.6865) -> (58.1603, 135.1865)
  line L520 (68.3205, 135.1865) -> (63.9904, 132.6865)
  line L521 (63.9904, 132.6865) -> (63.9904, 127.6865)
  line L522 (63.9904, 127.6865) -> (68.3205, 125.1865)
  line L523 (68.3205, 125.1865) -> (72.6506, 127.6865)
  line L524 (72.6506, 127.6865) -> (72.6506, 132.6865)
  line L525 (72.6506, 132.6865) -> (68.3205, 135.1865)
  line L526 (78.4808, 135.1865) -> (74.1506, 132.6865)
  line L527 (74.1506, 132.6865) -> (74.1506, 127.6865)
  line L528 (74.1506, 127.6865) -> (78.4808, 125.1865)
  line L529 (78.4808, 125.1865) -> (82.8109, 127.6865)
  line L530 (82.8109, 127.6865) -> (82.8109, 132.6865)
  line L531 (82.8109, 132.6865) -> (78.4808, 135.1865)
  line L532 (88.641, 135.1865) -> (84.3109, 132.6865)
  line L533 (84.3109, 132.6865) -> (84.3109, 127.6865)
  line L534 (84.3109, 127.6865) -> (88.641, 125.1865)
  line L535 (88.641, 125.1865) -> (92.9711, 127.6865)
  line L536 (92.9711, 127.6865) -> (92.9711, 132.6865)
  line L537 (92.9711, 132.6865) -> (88.641, 135.1865)
  line L538 (98.8013, 135.1865) -> (94.4711, 132.6865)
  line L539 (94.4711, 132.6865) -> (94.4711, 127.6865)
  line L540 (94.4711, 127.6865) -> (98.8013, 125.1865)
  line L541 (98.8013, 125.1865) -> (103.1314, 127.6865)
  line L542 (103.1314, 127.6865) -> (103.1314, 132.6865)
  line L543 (103.1314, 132.6865) -> (98.8013, 135.1865)
  line L544 (108.9615, 135.1865) -> (104.6314, 132.6865)
  line L545 (104.6314, 132.6865) -> (104.6314, 127.6865)
  line L546 (104.6314, 127.6865) -> (108.9615, 125.1865)
  line L547 (108.9615, 125.1865) -> (113.2917, 127.6865)
  line L548 (113.2917, 127.6865) -> (113.2917, 132.6865)
  line L549 (113.2917, 132.6865) -> (108.9615, 135.1865)
extrude "拉伸25" cut sketch "草图25" against normal blind 5 contours L4 L5 L6 L7 L8 L9 | L10 L11 L12 L13 L14 L15 | L16 L17 L18 L19 L20 L21 | L22 L23 L24 L25 L26 L27 | L28 L29 L30 L31 L32 L33 | L34 L35 L36 L37 L38 L39 | L40 L41 L42 L43 L44 L45 | L46 L47 L48 L49 L50 L51 | L52 L53 L54 L55 L56 L57 | L58 L59 L60 L61 L62 L63 | L64 L65 L66 L67 L68 L69 | L70 L71 L72 L73 L74 L75 | L76 L77 L78 L79 L80 L81 | L82 L83 L84 L85 L86 L87 | L88 L89 L90 L91 L92 L93 | L94 L95 L96 L97 L98 L99 | L100 L101 L102 L103 L104 L105 | L106 L107 L108 L109 L110 L111 | L112 L113 L114 L115 L116 L117 | L118 L119 L120 L121 L122 L123 | L124 L125 L126 L127 L128 L129 | L130 L131 L132 L133 L134 L135 | L136 L137 L138 L139 L140 L141 | L142 L143 L144 L145 L146 L147 | L148 L149 L150 L151 L152 L153 | L154 L155 L156 L157 L158 L159 | L160 L161 L162 L163 L164 L165 | L166 L167 L168 L169 L170 L171 | L172 L173 L174 L175 L176 L177 | L178 L179 L180 L181 L182 L183 | L184 L185 L186 L187 L188 L189 | L190 L191 L192 L193 L194 L195 | L196 L197 L198 L199 L200 L201 | L202 L203 L204 L205 L206 L207 | L208 L209 L210 L211 L212 L213 | L214 L215 L216 L217 L218 L219 | L220 L221 L222 L223 L224 L225 | L226 L227 L228 L229 L230 L231 | L232 L233 L234 L235 L236 L237 | L238 L239 L240 L241 L242 L243 | L244 L245 L246 L247 L248 L249 | L250 L251 L252 L253 L254 L255 | L256 L257 L258 L259 L260 L261 | L262 L263 L264 L265 L266 L267 | L268 L269 L270 L271 L272 L273 | L274 L275 L276 L277 L278 L279 | L280 L281 L282 L283 L284 L285 | L286 L287 L288 L289 L290 L291 | L292 L293 L294 L295 L296 L297 | L298 L299 L300 L301 L302 L303 | L304 L305 L306 L307 L308 L309 | L310 L311 L312 L313 L314 L315 | L316 L317 L318 L319 L320 L321 | L322 L323 L324 L325 L326 L327 | L328 L329 L330 L331 L332 L333 | L334 L335 L336 L337 L338 L339 | L340 L341 L342 L343 L344 L345 | L346 L347 L348 L349 L350 L351 | L352 L353 L354 L355 L356 L357 | L358 L359 L360 L361 L362 L363 | L364 L365 L366 L367 L368 L369 | L370 L371 L372 L373 L374 L375 | L376 L377 L378 L379 L380 L381 | L382 L383 L384 L385 L386 L387 | L388 L389 L390 L391 L392 L393 | L394 L395 L396 L397 L398 L399 | L400 L401 L402 L403 L404 L405 | L406 L407 L408 L409 L410 L411 | L412 L413 L414 L415 L416 L417 | L418 L419 L420 L421 L422 L423 | L424 L425 L426 L427 L428 L429 | L430 L431 L432 L433 L434 L435 | L436 L437 L438 L439 L440 L441 | L442 L443 L444 L445 L446 L447 | L448 L449 L450 L451 L452 L453 | L454 L455 L456 L457 L458 L459 | L460 L461 L462 L463 L464 L465 | L466 L467 L468 L469 L470 L471 | L472 L473 L474 L475 L476 L477 | L478 L479 L480 L481 L482 L483 | L484 L485 L486 L487 L488 L489 | L490 L491 L492 L493 L494 L495 | L496 L497 L498 L499 L500 L501 | L502 L503 L504 L505 L506 L507 | L508 L509 L510 L511 L512 L513 | L514 L515 L516 L517 L518 L519 | L520 L521 L522 L523 L524 L525 | L526 L527 L528 L529 L530 L531 | L532 L533 L534 L535 L536 L537 | L538 L539 L540 L541 L542 L543 | L544 L545 L546 L547 L548 L549 bodies 1 3
sketch "草图26" plane through (0, -116, 0) normal (0, 1, 0) x (-1, 0, 0)
  line L0 (-116, 0) -> (-7, 0)
  line L1 (-7, 0) -> (-7, 120)
  line L2 (-7, 120) -> (-116, 120)
  line L3 (-116, 120) -> (-116, 0)
  line L4 (-103.9199, 20.799) -> (-108.25, 18.299)
  line L5 (-108.25, 18.299) -> (-108.25, 13.299)
  line L6 (-108.25, 13.299) -> (-103.9199, 10.799)
  line L7 (-103.9199, 10.799) -> (-99.5897, 13.299)
  line L8 (-99.5897, 13.299) -> (-99.5897, 18.299)
  line L9 (-99.5897, 18.299) -> (-103.9199, 20.799)
  line L10 (-93.7596, 20.799) -> (-98.0897, 18.299)
  line L11 (-98.0897, 18.299) -> (-98.0897, 13.299)
  line L12 (-98.0897, 13.299) -> (-93.7596, 10.799)
  line L13 (-93.7596, 10.799) -> (-89.4295, 13.299)
  line L14 (-89.4295, 13.299) -> (-89.4295, 18.299)
  line L15 (-89.4295, 18.299) -> (-93.7596, 20.799)
  line L16 (-83.5994, 20.799) -> (-87.9295, 18.299)
  line L17 (-87.9295, 18.299) -> (-87.9295, 13.299)
  line L18 (-87.9295, 13.299) -> (-83.5994, 10.799)
  line L19 (-83.5994, 10.799) -> (-79.2692, 13.299)
  line L20 (-79.2692, 13.299) -> (-79.2692, 18.299)
  line L21 (-79.2692, 18.299) -> (-83.5994, 20.799)
  line L22 (-73.4391, 20.799) -> (-77.7692, 18.299)
  line L23 (-77.7692, 18.299) -> (-77.7692, 13.299)
  line L24 (-77.7692, 13.299) -> (-73.4391, 10.799)
  line L25 (-73.4391, 10.799) -> (-69.109, 13.299)
  line L26 (-69.109, 13.299) -> (-69.109, 18.299)
  line L27 (-69.109, 18.299) -> (-73.4391, 20.799)
  line L28 (-63.2789, 20.799) -> (-67.609, 18.299)
  line L29 (-67.609, 18.299) -> (-67.609, 13.299)
  line L30 (-67.609, 13.299) -> (-63.2789, 10.799)
  line L31 (-63.2789, 10.799) -> (-58.9487, 13.299)
  line L32 (-58.9487, 13.299) -> (-58.9487, 18.299)
  line L33 (-58.9487, 18.299) -> (-63.2789, 20.799)
  line L34 (-53.1186, 20.799) -> (-57.4487, 18.299)
  line L35 (-57.4487, 18.299) -> (-57.4487, 13.299)
  line L36 (-57.4487, 13.299) -> (-53.1186, 10.799)
  line L37 (-53.1186, 10.799) -> (-48.7885, 13.299)
  line L38 (-48.7885, 13.299) -> (-48.7885, 18.299)
  line L39 (-48.7885, 18.299) -> (-53.1186, 20.799)
  line L40 (-42.9583, 20.799) -> (-47.2885, 18.299)
  line L41 (-47.2885, 18.299) -> (-47.2885, 13.299)
  line L42 (-47.2885, 13.299) -> (-42.9583, 10.799)
  line L43 (-42.9583, 10.799) -> (-38.6282, 13.299)
  line L44 (-38.6282, 13.299) -> (-38.6282, 18.299)
  line L45 (-38.6282, 18.299) -> (-42.9583, 20.799)
  line L46 (-32.7981, 20.799) -> (-37.1282, 18.299)
  line L47 (-37.1282, 18.299) -> (-37.1282, 13.299)
  line L48 (-37.1282, 13.299) -> (-32.7981, 10.799)
  line L49 (-32.7981, 10.799) -> (-28.468, 13.299)
  line L50 (-28.468, 13.299) -> (-28.468, 18.299)
  line L51 (-28.468, 18.299) -> (-32.7981, 20.799)
  line L52 (-22.6378, 20.799) -> (-26.968, 18.299)
  line L53 (-26.968, 18.299) -> (-26.968, 13.299)
  line L54 (-26.968, 13.299) -> (-22.6378, 10.799)
  line L55 (-22.6378, 10.799) -> (-18.3077, 13.299)
  line L56 (-18.3077, 13.299) -> (-18.3077, 18.299)
  line L57 (-18.3077, 18.299) -> (-22.6378, 20.799)
  line L58 (-109, 29.5981) -> (-113.3301, 27.0981)
  line L59 (-113.3301, 27.0981) -> (-113.3301, 22.0981)
  line L60 (-113.3301, 22.0981) -> (-109, 19.5981)
  line L61 (-109, 19.5981) -> (-104.6699, 22.0981)
  line L62 (-104.6699, 22.0981) -> (-104.6699, 27.0981)
  line L63 (-104.6699, 27.0981) -> (-109, 29.5981)
  line L64 (-98.8397, 29.5981) -> (-103.1699, 27.0981)
  line L65 (-103.1699, 27.0981) -> (-103.1699, 22.0981)
  line L66 (-103.1699, 22.0981) -> (-98.8397, 19.5981)
  line L67 (-98.8397, 19.5981) -> (-94.5096, 22.0981)
  line L68 (-94.5096, 22.0981) -> (-94.5096, 27.0981)
  line L69 (-94.5096, 27.0981) -> (-98.8397, 29.5981)
  line L70 (-88.6795, 29.5981) -> (-93.0096, 27.0981)
  line L71 (-93.0096, 27.0981) -> (-93.0096, 22.0981)
  line L72 (-93.0096, 22.0981) -> (-88.6795, 19.5981)
  line L73 (-88.6795, 19.5981) -> (-84.3494, 22.0981)
  line L74 (-84.3494, 22.0981) -> (-84.3494, 27.0981)
  line L75 (-84.3494, 27.0981) -> (-88.6795, 29.5981)
  line L76 (-78.5192, 29.5981) -> (-82.8494, 27.0981)
  line L77 (-82.8494, 27.0981) -> (-82.8494, 22.0981)
  line L78 (-82.8494, 22.0981) -> (-78.5192, 19.5981)
  line L79 (-78.5192, 19.5981) -> (-74.1891, 22.0981)
  line L80 (-74.1891, 22.0981) -> (-74.1891, 27.0981)
  line L81 (-74.1891, 27.0981) -> (-78.5192, 29.5981)
  line L82 (-68.359, 29.5981) -> (-72.6891, 27.0981)
  line L83 (-72.6891, 27.0981) -> (-72.6891, 22.0981)
  line L84 (-72.6891, 22.0981) -> (-68.359, 19.5981)
  line L85 (-68.359, 19.5981) -> (-64.0289, 22.0981)
  line L86 (-64.0289, 22.0981) -> (-64.0289, 27.0981)
  line L87 (-64.0289, 27.0981) -> (-68.359, 29.5981)
  line L88 (-58.1987, 29.5981) -> (-62.5289, 27.0981)
  line L89 (-62.5289, 27.0981) -> (-62.5289, 22.0981)
  line L90 (-62.5289, 22.0981) -> (-58.1987, 19.5981)
  line L91 (-58.1987, 19.5981) -> (-53.8686, 22.0981)
  line L92 (-53.8686, 22.0981) -> (-53.8686, 27.0981)
  line L93 (-53.8686, 27.0981) -> (-58.1987, 29.5981)
  line L94 (-48.0385, 29.5981) -> (-52.3686, 27.0981)
  line L95 (-52.3686, 27.0981) -> (-52.3686, 22.0981)
  line L96 (-52.3686, 22.0981) -> (-48.0385, 19.5981)
  line L97 (-48.0385, 19.5981) -> (-43.7083, 22.0981)
  line L98 (-43.7083, 22.0981) -> (-43.7083, 27.0981)
  line L99 (-43.7083, 27.0981) -> (-48.0385, 29.5981)
  line L100 (-37.8782, 29.5981) -> (-42.2083, 27.0981)
  line L101 (-42.2083, 27.0981) -> (-42.2083, 22.0981)
  line L102 (-42.2083, 22.0981) -> (-37.8782, 19.5981)
  line L103 (-37.8782, 19.5981) -> (-33.5481, 22.0981)
  line L104 (-33.5481, 22.0981) -> (-33.5481, 27.0981)
  line L105 (-33.5481, 27.0981) -> (-37.8782, 29.5981)
  line L106 (-27.718, 29.5981) -> (-32.0481, 27.0981)
  line L107 (-32.0481, 27.0981) -> (-32.0481, 22.0981)
  line L108 (-32.0481, 22.0981) -> (-27.718, 19.5981)
  line L109 (-27.718, 19.5981) -> (-23.3878, 22.0981)
  line L110 (-23.3878, 22.0981) -> (-23.3878, 27.0981)
  line L111 (-23.3878, 27.0981) -> (-27.718, 29.5981)
  line L112 (-17.5577, 29.5981) -> (-21.8878, 27.0981)
  line L113 (-21.8878, 27.0981) -> (-21.8878, 22.0981)
  line L114 (-21.8878, 22.0981) -> (-17.5577, 19.5981)
  line L115 (-17.5577, 19.5981) -> (-13.2276, 22.0981)
  line L116 (-13.2276, 22.0981) -> (-13.2276, 27.0981)
  line L117 (-13.2276, 27.0981) -> (-17.5577, 29.5981)
  line L118 (-103.9199, 38.3971) -> (-108.25, 35.8971)
  line L119 (-108.25, 35.8971) -> (-108.25, 30.8971)
  line L120 (-108.25, 30.8971) -> (-103.9199, 28.3971)
  line L121 (-103.9199, 28.3971) -> (-99.5897, 30.8971)
  line L122 (-99.5897, 30.8971) -> (-99.5897, 35.8971)
  line L123 (-99.5897, 35.8971) -> (-103.9199, 38.3971)
  line L124 (-93.7596, 38.3971) -> (-98.0897, 35.8971)
  line L125 (-98.0897, 35.8971) -> (-98.0897, 30.8971)
  line L126 (-98.0897, 30.8971) -> (-93.7596, 28.3971)
  line L127 (-93.7596, 28.3971) -> (-89.4295, 30.8971)
  line L128 (-89.4295, 30.8971) -> (-89.4295, 35.8971)
  line L129 (-89.4295, 35.8971) -> (-93.7596, 38.3971)
  line L130 (-83.5994, 38.3971) -> (-87.9295, 35.8971)
  line L131 (-87.9295, 35.8971) -> (-87.9295, 30.8971)
  line L132 (-87.9295, 30.8971) -> (-83.5994, 28.3971)
  line L133 (-83.5994, 28.3971) -> (-79.2692, 30.8971)
  line L134 (-79.2692, 30.8971) -> (-79.2692, 35.8971)
  line L135 (-79.2692, 35.8971) -> (-83.5994, 38.3971)
  line L136 (-73.4391, 38.3971) -> (-77.7692, 35.8971)
  line L137 (-77.7692, 35.8971) -> (-77.7692, 30.8971)
  line L138 (-77.7692, 30.8971) -> (-73.4391, 28.3971)
  line L139 (-73.4391, 28.3971) -> (-69.109, 30.8971)
  line L140 (-69.109, 30.8971) -> (-69.109, 35.8971)
  line L141 (-69.109, 35.8971) -> (-73.4391, 38.3971)
  line L142 (-63.2789, 38.3971) -> (-67.609, 35.8971)
  line L143 (-67.609, 35.8971) -> (-67.609, 30.8971)
  line L144 (-67.609, 30.8971) -> (-63.2789, 28.3971)
  line L145 (-63.2789, 28.3971) -> (-58.9487, 30.8971)
  line L146 (-58.9487, 30.8971) -> (-58.9487, 35.8971)
  line L147 (-58.9487, 35.8971) -> (-63.2789, 38.3971)
  line L148 (-53.1186, 38.3971) -> (-57.4487, 35.8971)
  line L149 (-57.4487, 35.8971) -> (-57.4487, 30.8971)
  line L150 (-57.4487, 30.8971) -> (-53.1186, 28.3971)
  line L151 (-53.1186, 28.3971) -> (-48.7885, 30.8971)
  line L152 (-48.7885, 30.8971) -> (-48.7885, 35.8971)
  line L153 (-48.7885, 35.8971) -> (-53.1186, 38.3971)
  line L154 (-42.9583, 38.3971) -> (-47.2885, 35.8971)
  line L155 (-47.2885, 35.8971) -> (-47.2885, 30.8971)
  line L156 (-47.2885, 30.8971) -> (-42.9583, 28.3971)
  line L157 (-42.9583, 28.3971) -> (-38.6282, 30.8971)
  line L158 (-38.6282, 30.8971) -> (-38.6282, 35.8971)
  line L159 (-38.6282, 35.8971) -> (-42.9583, 38.3971)
  line L160 (-32.7981, 38.3971) -> (-37.1282, 35.8971)
  line L161 (-37.1282, 35.8971) -> (-37.1282, 30.8971)
  line L162 (-37.1282, 30.8971) -> (-32.7981, 28.3971)
  line L163 (-32.7981, 28.3971) -> (-28.468, 30.8971)
  line L164 (-28.468, 30.8971) -> (-28.468, 35.8971)
  line L165 (-28.468, 35.8971) -> (-32.7981, 38.3971)
  line L166 (-22.6378, 38.3971) -> (-26.968, 35.8971)
  line L167 (-26.968, 35.8971) -> (-26.968, 30.8971)
  line L168 (-26.968, 30.8971) -> (-22.6378, 28.3971)
  line L169 (-22.6378, 28.3971) -> (-18.3077, 30.8971)
  line L170 (-18.3077, 30.8971) -> (-18.3077, 35.8971)
  line L171 (-18.3077, 35.8971) -> (-22.6378, 38.3971)
  line L172 (-109, 47.1962) -> (-113.3301, 44.6962)
  line L173 (-113.3301, 44.6962) -> (-113.3301, 39.6962)
  line L174 (-113.3301, 39.6962) -> (-109, 37.1962)
  line L175 (-109, 37.1962) -> (-104.6699, 39.6962)
  line L176 (-104.6699, 39.6962) -> (-104.6699, 44.6962)
  line L177 (-104.6699, 44.6962) -> (-109, 47.1962)
  line L178 (-98.8397, 47.1962) -> (-103.1699, 44.6962)
  line L179 (-103.1699, 44.6962) -> (-103.1699, 39.6962)
  line L180 (-103.1699, 39.6962) -> (-98.8397, 37.1962)
  line L181 (-98.8397, 37.1962) -> (-94.5096, 39.6962)
  line L182 (-94.5096, 39.6962) -> (-94.5096, 44.6962)
  line L183 (-94.5096, 44.6962) -> (-98.8397, 47.1962)
  line L184 (-88.6795, 47.1962) -> (-93.0096, 44.6962)
  line L185 (-93.0096, 44.6962) -> (-93.0096, 39.6962)
  line L186 (-93.0096, 39.6962) -> (-88.6795, 37.1962)
  line L187 (-88.6795, 37.1962) -> (-84.3494, 39.6962)
  line L188 (-84.3494, 39.6962) -> (-84.3494, 44.6962)
  line L189 (-84.3494, 44.6962) -> (-88.6795, 47.1962)
  line L190 (-78.5192, 47.1962) -> (-82.8494, 44.6962)
  line L191 (-82.8494, 44.6962) -> (-82.8494, 39.6962)
  line L192 (-82.8494, 39.6962) -> (-78.5192, 37.1962)
  line L193 (-78.5192, 37.1962) -> (-74.1891, 39.6962)
  line L194 (-74.1891, 39.6962) -> (-74.1891, 44.6962)
  line L195 (-74.1891, 44.6962) -> (-78.5192, 47.1962)
  line L196 (-68.359, 47.1962) -> (-72.6891, 44.6962)
  line L197 (-72.6891, 44.6962) -> (-72.6891, 39.6962)
  line L198 (-72.6891, 39.6962) -> (-68.359, 37.1962)
  line L199 (-68.359, 37.1962) -> (-64.0289, 39.6962)
  line L200 (-64.0289, 39.6962) -> (-64.0289, 44.6962)
  line L201 (-64.0289, 44.6962) -> (-68.359, 47.1962)
  line L202 (-58.1987, 47.1962) -> (-62.5289, 44.6962)
  line L203 (-62.5289, 44.6962) -> (-62.5289, 39.6962)
  line L204 (-62.5289, 39.6962) -> (-58.1987, 37.1962)
  line L205 (-58.1987, 37.1962) -> (-53.8686, 39.6962)
  line L206 (-53.8686, 39.6962) -> (-53.8686, 44.6962)
  line L207 (-53.8686, 44.6962) -> (-58.1987, 47.1962)
  line L208 (-48.0385, 47.1962) -> (-52.3686, 44.6962)
  line L209 (-52.3686, 44.6962) -> (-52.3686, 39.6962)
  line L210 (-52.3686, 39.6962) -> (-48.0385, 37.1962)
  line L211 (-48.0385, 37.1962) -> (-43.7083, 39.6962)
  line L212 (-43.7083, 39.6962) -> (-43.7083, 44.6962)
  line L213 (-43.7083, 44.6962) -> (-48.0385, 47.1962)
  line L214 (-37.8782, 47.1962) -> (-42.2083, 44.6962)
  line L215 (-42.2083, 44.6962) -> (-42.2083, 39.6962)
  line L216 (-42.2083, 39.6962) -> (-37.8782, 37.1962)
  line L217 (-37.8782, 37.1962) -> (-33.5481, 39.6962)
  line L218 (-33.5481, 39.6962) -> (-33.5481, 44.6962)
  line L219 (-33.5481, 44.6962) -> (-37.8782, 47.1962)
  line L220 (-27.718, 47.1962) -> (-32.0481, 44.6962)
  line L221 (-32.0481, 44.6962) -> (-32.0481, 39.6962)
  line L222 (-32.0481, 39.6962) -> (-27.718, 37.1962)
  line L223 (-27.718, 37.1962) -> (-23.3878, 39.6962)
  line L224 (-23.3878, 39.6962) -> (-23.3878, 44.6962)
  line L225 (-23.3878, 44.6962) -> (-27.718, 47.1962)
  line L226 (-17.5577, 47.1962) -> (-21.8878, 44.6962)
  line L227 (-21.8878, 44.6962) -> (-21.8878, 39.6962)
  line L228 (-21.8878, 39.6962) -> (-17.5577, 37.1962)
  line L229 (-17.5577, 37.1962) -> (-13.2276, 39.6962)
  line L230 (-13.2276, 39.6962) -> (-13.2276, 44.6962)
  line L231 (-13.2276, 44.6962) -> (-17.5577, 47.1962)
  line L232 (-103.9199, 55.9952) -> (-108.25, 53.4952)
  line L233 (-108.25, 53.4952) -> (-108.25, 48.4952)
  line L234 (-108.25, 48.4952) -> (-103.9199, 45.9952)
  line L235 (-103.9199, 45.9952) -> (-99.5897, 48.4952)
  line L236 (-99.5897, 48.4952) -> (-99.5897, 53.4952)
  line L237 (-99.5897, 53.4952) -> (-103.9199, 55.9952)
  line L238 (-93.7596, 55.9952) -> (-98.0897, 53.4952)
  line L239 (-98.0897, 53.4952) -> (-98.0897, 48.4952)
  line L240 (-98.0897, 48.4952) -> (-93.7596, 45.9952)
  line L241 (-93.7596, 45.9952) -> (-89.4295, 48.4952)
  line L242 (-89.4295, 48.4952) -> (-89.4295, 53.4952)
  line L243 (-89.4295, 53.4952) -> (-93.7596, 55.9952)
  line L244 (-83.5994, 55.9952) -> (-87.9295, 53.4952)
  line L245 (-87.9295, 53.4952) -> (-87.9295, 48.4952)
  line L246 (-87.9295, 48.4952) -> (-83.5994, 45.9952)
  line L247 (-83.5994, 45.9952) -> (-79.2692, 48.4952)
  line L248 (-79.2692, 48.4952) -> (-79.2692, 53.4952)
  line L249 (-79.2692, 53.4952) -> (-83.5994, 55.9952)
  line L250 (-73.4391, 55.9952) -> (-77.7692, 53.4952)
  line L251 (-77.7692, 53.4952) -> (-77.7692, 48.4952)
  line L252 (-77.7692, 48.4952) -> (-73.4391, 45.9952)
  line L253 (-73.4391, 45.9952) -> (-69.109, 48.4952)
  line L254 (-69.109, 48.4952) -> (-69.109, 53.4952)
  line L255 (-69.109, 53.4952) -> (-73.4391, 55.9952)
  line L256 (-63.2789, 55.9952) -> (-67.609, 53.4952)
  line L257 (-67.609, 53.4952) -> (-67.609, 48.4952)
  line L258 (-67.609, 48.4952) -> (-63.2789, 45.9952)
  line L259 (-63.2789, 45.9952) -> (-58.9487, 48.4952)
  line L260 (-58.9487, 48.4952) -> (-58.9487, 53.4952)
  line L261 (-58.9487, 53.4952) -> (-63.2789, 55.9952)
  line L262 (-53.1186, 55.9952) -> (-57.4487, 53.4952)
  line L263 (-57.4487, 53.4952) -> (-57.4487, 48.4952)
  line L264 (-57.4487, 48.4952) -> (-53.1186, 45.9952)
  line L265 (-53.1186, 45.9952) -> (-48.7885, 48.4952)
  line L266 (-48.7885, 48.4952) -> (-48.7885, 53.4952)
  line L267 (-48.7885, 53.4952) -> (-53.1186, 55.9952)
  line L268 (-42.9583, 55.9952) -> (-47.2885, 53.4952)
  line L269 (-47.2885, 53.4952) -> (-47.2885, 48.4952)
  line L270 (-47.2885, 48.4952) -> (-42.9583, 45.9952)
  line L271 (-42.9583, 45.9952) -> (-38.6282, 48.4952)
  line L272 (-38.6282, 48.4952) -> (-38.6282, 53.4952)
  line L273 (-38.6282, 53.4952) -> (-42.9583, 55.9952)
  line L274 (-32.7981, 55.9952) -> (-37.1282, 53.4952)
  line L275 (-37.1282, 53.4952) -> (-37.1282, 48.4952)
  line L276 (-37.1282, 48.4952) -> (-32.7981, 45.9952)
  line L277 (-32.7981, 45.9952) -> (-28.468, 48.4952)
  line L278 (-28.468, 48.4952) -> (-28.468, 53.4952)
  line L279 (-28.468, 53.4952) -> (-32.7981, 55.9952)
  line L280 (-22.6378, 55.9952) -> (-26.968, 53.4952)
  line L281 (-26.968, 53.4952) -> (-26.968, 48.4952)
  line L282 (-26.968, 48.4952) -> (-22.6378, 45.9952)
  line L283 (-22.6378, 45.9952) -> (-18.3077, 48.4952)
  line L284 (-18.3077, 48.4952) -> (-18.3077, 53.4952)
  line L285 (-18.3077, 53.4952) -> (-22.6378, 55.9952)
  line L286 (-109, 64.7942) -> (-113.3301, 62.2942)
  line L287 (-113.3301, 62.2942) -> (-113.3301, 57.2942)
  line L288 (-113.3301, 57.2942) -> (-109, 54.7942)
  line L289 (-109, 54.7942) -> (-104.6699, 57.2942)
  line L290 (-104.6699, 57.2942) -> (-104.6699, 62.2942)
  line L291 (-104.6699, 62.2942) -> (-109, 64.7942)
  line L292 (-98.8397, 64.7942) -> (-103.1699, 62.2942)
  line L293 (-103.1699, 62.2942) -> (-103.1699, 57.2942)
  line L294 (-103.1699, 57.2942) -> (-98.8397, 54.7942)
  line L295 (-98.8397, 54.7942) -> (-94.5096, 57.2942)
  line L296 (-94.5096, 57.2942) -> (-94.5096, 62.2942)
  line L297 (-94.5096, 62.2942) -> (-98.8397, 64.7942)
  line L298 (-88.6795, 64.7942) -> (-93.0096, 62.2942)
  line L299 (-93.0096, 62.2942) -> (-93.0096, 57.2942)
  line L300 (-93.0096, 57.2942) -> (-88.6795, 54.7942)
  line L301 (-88.6795, 54.7942) -> (-84.3494, 57.2942)
  line L302 (-84.3494, 57.2942) -> (-84.3494, 62.2942)
  line L303 (-84.3494, 62.2942) -> (-88.6795, 64.7942)
  line L304 (-78.5192, 64.7942) -> (-82.8494, 62.2942)
  line L305 (-82.8494, 62.2942) -> (-82.8494, 57.2942)
  line L306 (-82.8494, 57.2942) -> (-78.5192, 54.7942)
  line L307 (-78.5192, 54.7942) -> (-74.1891, 57.2942)
  line L308 (-74.1891, 57.2942) -> (-74.1891, 62.2942)
  line L309 (-74.1891, 62.2942) -> (-78.5192, 64.7942)
  line L310 (-68.359, 64.7942) -> (-72.6891, 62.2942)
  line L311 (-72.6891, 62.2942) -> (-72.6891, 57.2942)
  line L312 (-72.6891, 57.2942) -> (-68.359, 54.7942)
  line L313 (-68.359, 54.7942) -> (-64.0289, 57.2942)
  line L314 (-64.0289, 57.2942) -> (-64.0289, 62.2942)
  line L315 (-64.0289, 62.2942) -> (-68.359, 64.7942)
  line L316 (-58.1987, 64.7942) -> (-62.5289, 62.2942)
  line L317 (-62.5289, 62.2942) -> (-62.5289, 57.2942)
  line L318 (-62.5289, 57.2942) -> (-58.1987, 54.7942)
  line L319 (-58.1987, 54.7942) -> (-53.8686, 57.2942)
  line L320 (-53.8686, 57.2942) -> (-53.8686, 62.2942)
  line L321 (-53.8686, 62.2942) -> (-58.1987, 64.7942)
  line L322 (-48.0385, 64.7942) -> (-52.3686, 62.2942)
  line L323 (-52.3686, 62.2942) -> (-52.3686, 57.2942)
  line L324 (-52.3686, 57.2942) -> (-48.0385, 54.7942)
  line L325 (-48.0385, 54.7942) -> (-43.7083, 57.2942)
  line L326 (-43.7083, 57.2942) -> (-43.7083, 62.2942)
  line L327 (-43.7083, 62.2942) -> (-48.0385, 64.7942)
  line L328 (-37.8782, 64.7942) -> (-42.2083, 62.2942)
  line L329 (-42.2083, 62.2942) -> (-42.2083, 57.2942)